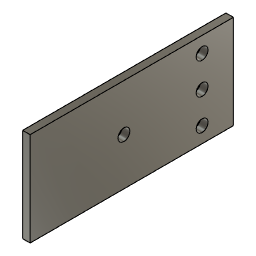
Elevator_BottomPlate v1 (Autodesk Fusion 360 design; units mm, degrees)
Autodesk Fusion 360 part; units mm, degrees
sketch "Sketch1" plane through (0, 0, 0) normal (1, 0, 0) x (0, 1, 0)
  line L0 (0, 0) -> (82.55, 0)
  line L1 (82.55, 0) -> (82.55, 38.1)
  line L2 (82.55, 38.1) -> (0, 38.1)
  line L3 (0, 38.1) -> (0, 0)
  dimension "d1" = 82.55
  dimension "d2" = 38.1
  constraint horizontal L0
  constraint vertical L1
  constraint horizontal L2
  constraint vertical L3
  constraint coincident L0.start L3.end
  measures "d1" distance of L0.start L0.end
  measures "d2" distance of L0.start L2.end
extrude "Extrude1" add sketch "Sketch1" along normal blind 3.048
sketch "Sketch2" plane through (3.048, 0, 0) normal (1, 0, 0) x (0, 1, 0)
  line L0 (0, 38.1) -> (0, 0)
  line L1 (0, 0) -> (82.55, 0)
  line L2 (82.55, 0) -> (82.55, 38.1)
  line L3 (82.55, 38.1) -> (0, 38.1)
  line L4 (0, 0) -> (38.1, 0)
  line L5 (38.1, 0) -> (38.1, 19.05)
  line L6 (38.1, 19.05) -> (0, 19.05)
  line L7 (0, 19.05) -> (0, 0)
  dimension "d5" = 38.1
  dimension "d6" = 19.05
  constraint horizontal L4
  constraint vertical L5
  constraint horizontal L6
  constraint vertical L7
  constraint coincident L0.end L1.start
  measures "d5" distance of L0.end L4.end
  measures "d6" distance of L0.end L6.end
hole "Hole1" at (3.048, 38.1, 19.05) direction (-1, 0, 0) diameter 4.826 depth 9.652 tip angle 118
sketch "Sketch3" plane through (3.048, 0, 0) normal (1, 0, 0) x (0, 1, 0)
  circle A0 centre (38.1, 19.05) radius 2.413
  line L0 (0, 38.1) -> (0, 0)
  line L1 (0, 0) -> (82.55, 0)
  line L2 (82.55, 0) -> (82.55, 38.1)
  line L3 (82.55, 38.1) -> (0, 38.1)
  line L4 (82.55, 0) -> (69.85, 0)
  line L5 (69.85, 0) -> (69.85, 6.35)
  line L6 (69.85, 6.35) -> (82.55, 6.35)
  line L7 (82.55, 6.35) -> (82.55, 0)
  dimension "d10" = 12.7
  dimension "d11" = 6.35
  constraint horizontal L4
  constraint vertical L5
  constraint horizontal L6
  constraint vertical L7
  constraint coincident L1.end L2.start
  measures "d10" distance of L1.end L4.end
  measures "d11" distance of L1.end L6.end
hole "Hole2" at (3.048, 69.85, 6.35) direction (-1, 0, 0) diameter 4.826 depth 3.048 tip angle 118
sketch "Sketch4" plane through (3.048, 0, 0) normal (1, 0, 0) x (0, 1, 0)
  circle A0 centre (69.85, 6.35) radius 2.413
  circle A1 centre (38.1, 19.05) radius 2.413
  line L0 (0, 38.1) -> (0, 0)
  line L1 (0, 0) -> (82.55, 0)
  line L2 (82.55, 0) -> (82.55, 38.1)
  line L3 (82.55, 38.1) -> (0, 38.1)
  line L4 (82.55, 0) -> (69.85, 0)
  line L5 (69.85, 0) -> (69.85, 19.05)
  line L6 (69.85, 19.05) -> (82.55, 19.05)
  line L7 (82.55, 19.05) -> (82.55, 0)
  dimension "d15" = 12.7
  dimension "d16" = 19.05
  constraint horizontal L4
  constraint vertical L5
  constraint horizontal L6
  constraint vertical L7
  constraint coincident L1.end L2.start
  measures "d15" distance of L1.end L4.end
  measures "d16" distance of L1.end L6.end
hole "Hole3" at (3.048, 69.85, 19.05) direction (-1, 0, 0) diameter 4.826 depth 3.048 tip angle 118
sketch "Sketch5" plane through (3.048, 0, 0) normal (1, 0, 0) x (0, 1, 0)
  circle A0 centre (69.85, 19.05) radius 2.413
  circle A1 centre (69.85, 6.35) radius 2.413
  circle A2 centre (38.1, 19.05) radius 2.413
  line L0 (0, 38.1) -> (0, 0)
  line L1 (0, 0) -> (82.55, 0)
  line L2 (82.55, 0) -> (82.55, 38.1)
  line L3 (82.55, 38.1) -> (0, 38.1)
  line L4 (82.55, 0) -> (69.85, 0)
  line L5 (69.85, 0) -> (69.85, 31.75)
  line L6 (69.85, 31.75) -> (82.55, 31.75)
  line L7 (82.55, 31.75) -> (82.55, 0)
  dimension "d20" = 12.7
  dimension "d21" = 31.75
  constraint horizontal L4
  constraint vertical L5
  constraint horizontal L6
  constraint vertical L7
  constraint coincident L1.end L2.start
  measures "d20" distance of L1.end L4.end
  measures "d21" distance of L1.end L6.end
hole "Hole4" at (3.048, 69.85, 31.75) direction (-1, 0, 0) diameter 4.826 depth 3.048 tip angle 118
